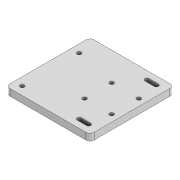
# Autodesk Inventor part: Electronics base
Saved by Autodesk Inventor 2020 (Build 240168000, 168)
## iProperties
Created: 2020-11-02
Part Number: Electronics base
Material: Generic
Document SubType Name: Modeling
Designer: ferrerx
Density: 1 g/cm^3
Appearance: Default
Author: ferrerx
Autodesk Inventor part; units mm, degrees
ref_plane "YZ Plane" through (0, 0, 0) normal (1, 0, 0) x (0, 1, 0)
ref_plane "XZ Plane" through (0, 0, 0) normal (0, 1, 0) x (-1, 0, 0)
ref_plane "XY Plane" through (0, 0, 0) normal (0, 0, 1) x (1, 0, 0)
sketch "Sketch1" plane through (0, 0, 0) normal (0, 1, 0) x (-1, 0, 0)
  line L0 (0, 0) -> (46, 0) construction
  line L1 (46, 0) -> (46, -46) construction
  line L2 (46, -46) -> (0, -46) construction
  line L3 (0, -46) -> (0, 0) construction
  circle A0 centre (46, -46) radius 1.5
  circle A1 centre (46, 0) radius 1.5
  circle A2 centre (0, 0) radius 1.5
  circle A3 centre (0, -46) radius 1.5
  line L4 (23, 0) -> (23, -46) construction
  line L5 (-8, 8) -> (54, 8)
  line L6 (54, 8) -> (54, -54)
  line L7 (54, -54) -> (-8, -54)
  line L8 (-8, -54) -> (-8, 8)
  line L9 (-8, 8) -> (54, -54) construction
  line L10 (54, 8) -> (-8, -54) construction
  point P0 (23, -23)
  dimension "d0" = 46
  dimension "d1" = 46
  dimension "d2" = 3
  dimension "d3" = 3
  dimension "d4" = 3
  dimension "d5" = 3
  dimension "d6" = 8
  dimension "d7" = 8
  constraints: 22 end point, 5 midpoint, 4 centre point, 4 coincident, 4 parallel, 2 horizontal, 2 perpendicular
  measures "d0" distance of L1.end L2.end
  measures "d1" distance of L2.end L0.start
  measures "d2" diameter of A0
  measures "d3" diameter of A1
  measures "d4" diameter of A2
  measures "d5" diameter of A3
  measures "d6" distance between parallel lines of L6 L1
  measures "d7" distance between parallel lines of L2 L7
extrude "Extrusion1" add sketch "Sketch1" along normal blind 5
sketch "Sketch2" plane through (0, 5, 0) normal (0, 1, 0) x (1, 0, 0)
  line L0 (-54, -8) -> (8, -8) projected
  line L1 (-54, -8) -> (-114, -8)
  line L2 (-114, -8) -> (-114, 54)
  line L3 (-114, 54) -> (-54, 54)
  line L4 (-54, 54) -> (-54, -8)
  line L5 (8, 54) -> (-54, 54) projected
  point P0 (0, 0)
  dimension "d10" = 60
  constraints: 8 end point, 2 parallel, 1 collinear, 1 horizontal, 1 perpendicular
  measures "d10" distance of L2.end L3.end
extrude "Extrusion2" add sketch "Sketch2" against normal blind 5
sketch "Sketch3" plane through (0, 5, 0) normal (0, 1, 0) x (1, 0, 0)
  circle A0 centre (0, 46) radius 1.5 projected
  circle A1 centre (-46, 46) radius 1.5 projected
  line L0 (0, 46) -> (-46, 46) construction
  line L1 (-23, 46) -> (-23, 0) construction
  line L2 (-1.5, 44.5) -> (-44.5, 44.5)
  line L3 (-44.5, 44.5) -> (-44.5, 1.5)
  line L4 (-44.5, 1.5) -> (-1.5, 1.5)
  line L5 (-1.5, 1.5) -> (-1.5, 44.5)
  line L6 (-1.5, 44.5) -> (-44.5, 1.5) construction
  line L7 (-44.5, 44.5) -> (-1.5, 1.5) construction
  line L8 (-114, -8) -> (8, -8) projected
  point P0 (0, 0)
  point P1 (-23, 23)
  dimension "d14" = 43
  dimension "d15" = 43
  constraints: 16 end point, 4 midpoint, 3 parallel, 1 horizontal, 1 perpendicular, 1 vertical
  measures "d14" distance of L2.start L2.end
  measures "d15" distance of L4.end L2.start
extrude "Extrusion3" cut sketch "Sketch3" against normal blind 5 contours L5 L4 L3 L2
fillet "Fillet1" radius 1 4 edges at (-44.5, 2.5, -44.5) (-44.5, 2.5, -1.5) (-1.5, 2.5, -1.5) (-1.5, 2.5, -44.5)
sketch "Sketch4" plane through (0, 5, 0) normal (0, 1, 0) x (1, 0, 0)
  circle A0 centre (-108, 40) radius 1.5
  circle A1 centre (-108, -2) radius 1.5
  line L0 (-114, -8) -> (8, -8) projected
  line L1 (-114, 54) -> (-114, -8) projected
  line L2 (8, 54) -> (-114, 54) projected
  circle A2 centre (-59, -2) radius 1.5
  circle A3 centre (-59, 48) radius 1.5
  circle A4 centre (-66, -2) radius 1.5
  circle A5 centre (-66, 48) radius 1.5
  line L3 (-59, -2) -> (-59, 48) construction
  line L4 (-66, 46.5) -> (-59, 46.5)
  line L5 (-66, 49.5) -> (-59, 49.5)
  line L6 (-66, -3.5) -> (-59, -3.5)
  line L7 (-66, -0.5) -> (-59, -0.5)
  line L8 (-66, -2) -> (-66, 48) construction
  line L9 (-59, -2) -> (-66, -2) construction
  line L10 (-59, 48) -> (-66, 48) construction
  point P0 (0, 0)
  dimension "d19" = 6
  dimension "d20" = 3
  dimension "d21" = 6
  dimension "d23" = 3
  dimension "d24" = 6
  dimension "d25" = 14
  dimension "d26" = 3
  dimension "d27" = 3
  dimension "d28" = 50
  dimension "d29" = 6
  dimension "d32" = 7
  dimension "d33" = 3
  dimension "d34" = 3
  dimension "d35" = 7
  dimension "d36" = 42
  constraints: 16 end point, 8 point on circle, 6 centre point, 3 horizontal, 2 point on line, 1 perpendicular, 1 tangent, 1 vertical
  measures "d19" distance from line of L0 A1.centre
  measures "d20" diameter of A1
  measures "d21" distance from line of L1 A1.centre
  measures "d23" diameter of A0
  measures "d24" distance from line of L1 A0.centre
  measures "d25" distance from line of L2 A0.centre
  measures "d26" diameter of A3
  measures "d27" diameter of A2
  measures "d28" distance of L3.end L3.start
  measures "d29" distance from line of L2 L3.end
  measures "d32" distance of L8.start L3.start
  measures "d33" diameter of A4
  measures "d34" diameter of A5
  measures "d35" distance of L8.end L3.end
  measures "d36" distance from line of A0.centre L8
extrude "Extrusion4" cut sketch "Sketch4" against normal blind 5
fillet "Fillet2" radius 3 4 edges at (8, 2.5, -54) (8, 2.5, 8) (-114, 2.5, 8) (-114, 2.5, -54)
sketch "Sketch5" plane through (0, 5, 0) normal (0, 1, 0) x (1, 0, 0)
  line L0 (-52, 54) -> (8, 54)
  line L1 (8, 54) -> (8, -8)
  line L2 (8, -8) -> (-52, -8)
  line L3 (-52, -8) -> (-52, 54)
  point P0 (0, 0)
  constraints: 8 end point, 2 parallel, 1 horizontal, 1 perpendicular
extrude "Extrusion5" cut sketch "Sketch5" against normal blind 10
fillet "Fillet3" radius 3 2 edges at (-52, 2.5, 8) (-52, 2.5, -54)
sketch "Sketch6" plane through (0, 5, 0) normal (0, 1, 0) x (1, 0, 0)
  line L0 (-52, 51) -> (-52, -5) projected
  line L1 (-52, 23) -> (-67, 23) construction
  line L2 (-77, 33) -> (-57, 33) construction
  line L3 (-57, 33) -> (-57, 13) construction
  line L4 (-57, 13) -> (-77, 13) construction
  line L5 (-77, 13) -> (-77, 33) construction
  line L6 (-77, 33) -> (-57, 13) construction
  line L7 (-57, 33) -> (-77, 13) construction
  circle A0 centre (-57, 33) radius 1.5
  circle A1 centre (-57, 13) radius 1.5
  circle A2 centre (-77, 13) radius 1.5
  circle A3 centre (-77, 33) radius 1.5
  point P0 (0, 0)
  dimension "d44" = 20
  dimension "d45" = 20
  dimension "d46" = 5
  dimension "d47" = 3
  dimension "d48" = 3
  dimension "d49" = 3
  dimension "d50" = 3
  constraints: 14 end point, 4 centre point, 4 coincident, 3 midpoint, 2 horizontal, 2 parallel, 1 perpendicular
  measures "d44" distance of L3.end L4.end
  measures "d45" distance of L4.end L2.start
  measures "d46" distance between parallel lines of L0 L3
  measures "d47" diameter of A0
  measures "d48" diameter of A1
  measures "d49" diameter of A2
  measures "d50" diameter of A3
extrude "Extrusion6" cut sketch "Sketch6" against normal blind 10
body "Solid1"
